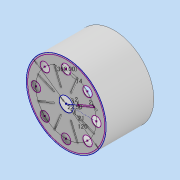
# Autodesk Inventor part: motorheadcoverouterEne1-1
Saved by Autodesk Inventor 2022 (Build 260153000, 153)
## iProperties
Created: 2024-05-03
Part Number: motorheadcoverouterEne1-1
Material: 一般
Document SubType Name: Modeling
Designer: ktamu
Density: 1 g/cm^3
Appearance: 既定
Author: ktamu
Autodesk Inventor part; units mm, degrees
ref_plane "YZ Plane" through (0, 0, 0) normal (1, 0, 0) x (0, 1, 0)
ref_plane "XZ Plane" through (0, 0, 0) normal (0, 1, 0) x (-1, 0, 0)
ref_plane "XY Plane" through (0, 0, 0) normal (0, 0, 1) x (1, 0, 0)
sketch "BASEsc" plane through (0, 0, 0) normal (0, 0, 1) x (1, 0, 0)
  circle A0 centre (0, 0) radius 58
  circle A1 centre (0, 0) radius 60
  circle A2 centre (0, 0) radius 10.5
  circle A3 centre (0, 45.4403) radius 7
  circle A4 centre (-32.1311, 32.1311) radius 7
  circle A5 centre (-45.4403, 0) radius 7
  circle A6 centre (-32.1311, -32.1311) radius 7
  circle A7 centre (0, -45.4403) radius 7
  circle A8 centre (32.1311, -32.1311) radius 7
  circle A9 centre (45.4403, 0) radius 7
  circle A10 centre (32.1311, 32.1311) radius 7
  line L0 (0, 0) -> (17.3018, 7.1667)
  line L1 (0, 0) -> (45.4403, 0) construction
  arc A11 (42.364, 16.4654) -> (41.5987, 18.3131) centre (41.9813, 17.3892) ccw
  arc A12 (17.843, 8.4732) -> (18.6084, 6.6255) centre (18.2257, 7.5493) ccw
  line L2 (42.364, 16.4654) -> (18.6084, 6.6255)
  line L3 (17.843, 8.4732) -> (41.5987, 18.3131)
  dimension "d1" = 120
  dimension "d2" = 21
  dimension "d3" = 14
  dimension "d6" = 360
  dimension "d18" = 22.5
  dimension "d19" = 2
  dimension "d20" = 2
  constraints: 13 centre point, 8 end point, 5 point on circle, 3 coincident, 1 horizontal, 1 parallel, 1 point on line, 17 other
  measures "d1" diameter of A1
  measures "d2" diameter of A2
  measures "d3" diameter of A3
  measures "d18" angle of L1 L0
  measures "d19" diameter of A11
  measures "d20" diameter of A12
extrude "押し出し1" add sketch "BASEsc" against normal blind 2 contours A0 | L2 A12 L3 A11
extrude "押し出し2" add sketch "BASEsc" against normal blind 72 contours A1
fillet "フィレット1" radius 1.5 9 edges at (-39.1311, -32.1311, -2) (-7, -45.4403, -2) (25.1311, -32.1311, -2) (-10.5, 0, -2) (-52.4403, 0, -2) (-39.1311, 32.1311, -2) (38.4403, 0, -2) (25.1311, 32.1311, -2) (-7, 45.4403, -2)
extrude "押し出し3" cut sketch "BASEsc" against normal through all contours L2 A12 L3 A11
pattern_circular "円形状パターン1" count 8 over 360 about axis through (0, 0, -0.5) along (0, 0, 1) of "押し出し3"
fillet "フィレット2" radius 0.5 32 edges at (17.3018, 7.1667, -2) (30.4862, 11.5454, -2) (42.9052, 17.7719, -2) (29.7208, 13.3932, -2) (17.7719, 42.9052, -2) (11.5454, 30.4862, -2) (7.1667, 17.3018, -2) (13.3932, 29.7208, -2) (-17.7719, 42.9052, -2) (-13.3932, 29.7208, -2) (-7.1667, 17.3018, -2) (-11.5454, 30.4862, -2) (-42.9052, 17.7719, -2) (-30.4862, 11.5454, -2) (-17.3018, 7.1667, -2) (-29.7208, 13.3932, -2) (-42.9052, -17.7719, -2) (-29.7208, -13.3932, -2) (-17.3018, -7.1667, -2) (-30.4862, -11.5454, -2) (-17.7719, -42.9052, -2) (-11.5454, -30.4862, -2) (-7.1667, -17.3018, -2) (-13.3932, -29.7208, -2) (17.7719, -42.9052, -2) (13.3932, -29.7208, -2) (7.1667, -17.3018, -2) (11.5454, -30.4862, -2) (42.9052, -17.7719, -2) (30.4862, -11.5454, -2) (17.3018, -7.1667, -2) (29.7208, -13.3932, -2)
